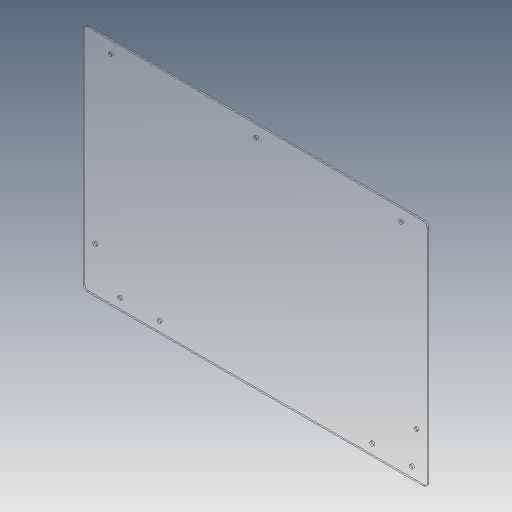
# Autodesk Inventor part: 防水2
Saved by Autodesk Inventor 2020.3 (Build 243373000, 373)
## iProperties
Part Number: 防水2
Material: PET プラスチック
Document SubType Name: Modeling
Designer: highs
Density: 1.541 g/cm^3
Appearance: ポリカーボネート - クリア
Author: highs
Autodesk Inventor part; units mm, degrees
ref_plane "YZ Plane" through (0, 0, 0) normal (1, 0, 0) x (0, 1, 0)
ref_plane "XZ Plane" through (0, 0, 0) normal (0, 1, 0) x (-1, 0, 0)
ref_plane "XY Plane" through (0, 0, 0) normal (0, 0, 1) x (1, 0, 0)
sketch "スケッチ1" plane through (0, 0, 0) normal (0, 0, 1) x (1, 0, 0)
  line L0 (0, 0) -> (450, 0)
  line L1 (450, 0) -> (450, 300)
  line L2 (450, 300) -> (0, 300)
  line L3 (0, 300) -> (0, 0)
  line L4 (435, 285) -> (435, 15) construction
  line L5 (435, 15) -> (15, 15) construction
  line L6 (15, 15) -> (15, 285) construction
  circle A0 centre (35, 284) radius 2.5
  circle A1 centre (415, 284) radius 2.5
  circle A2 centre (225, 284) radius 2.5
  circle A3 centre (47, 13.6) radius 2.5
  circle A4 centre (99, 13.6) radius 2.5
  line L7 (47, 13.6) -> (99, 13.6) construction
  circle A5 centre (429, 13.6) radius 2.5
  circle A6 centre (377, 13.6) radius 2.5
  line L8 (429, 13.6) -> (377, 13.6) construction
  line L9 (225, 0) -> (225, 15) construction
  circle A7 centre (435, 59) radius 2.5
  circle A8 centre (15, 59) radius 2.5
  line L10 (35, 284) -> (415, 284) construction
  dimension "d0" = 450
  dimension "d1" = 300
  dimension "d3" = 35
  dimension "d4" = 35
  dimension "d5" = 5
  dimension "d8" = 13.6
  dimension "d9" = 5
  dimension "d10" = 47
  dimension "d11" = 52
  dimension "d12" = 21
  dimension "d13" = 13.6
  dimension "d14" = 52
  dimension "d19" = 16
  dimension "d20" = 59
  dimension "d21" = 59
  dimension "d22" = 15
  constraints: 22 end point, 9 centre point, 7 equal radius, 3 horizontal, 3 midpoint, 3 parallel, 2 perpendicular, 2 point on line, 2 other
  measures "d0" distance of L0.start L0.end
  measures "d1" distance of L2.end L0.start
  measures "d3" distance from line of L3 L10.start
  measures "d4" distance from line of L1 L10.end
  measures "d5" diameter of A0
  measures "d8" distance from line of L0 L7.start
  measures "d9" diameter of A3
  measures "d10" distance from line of L3 L7.start
  measures "d11" distance of L7.start L7.end
  measures "d12" distance from line of L1 L8.start
  measures "d13" distance between parallel lines of L0 L8
  measures "d14" distance of L8.start L8.end
  measures "d19" distance between parallel lines of L2 L10
  measures "d20" distance from line of L0 A8.centre
  measures "d21" distance from line of L0 A7.centre
  measures "d22" distance from line of L3 A8.centre
extrude "押し出し1" add sketch "スケッチ1" along normal blind 2
fillet "フィレット1" radius 5 4 edges at (450, 0, 1) (450, 300, 1) (0, 0, 1) (0, 300, 1)
